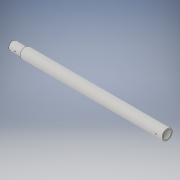
# Autodesk Inventor part: 1_6RadiusPoleAJB
Saved by Autodesk Inventor 2018 (Build 220112000, 112)
## iProperties
Created: 2018-02-02
Part Number: 1_6RadiusPoleAJB
Material: Generic
Document SubType Name: Modeling
Designer: Alec temporary
Density: 1 g/cm^3
Appearance: Default
Author: Alec temporary
Autodesk Inventor part; units mm, degrees
ref_plane "YZ Plane" through (0, 0, 0) normal (1, 0, 0) x (0, 1, 0)
ref_plane "XZ Plane" through (0, 0, 0) normal (0, 1, 0) x (-1, 0, 0)
sketch "Sketch1" plane through (0, 0, 0) normal (0, 0, 1) x (1, 0, 0)
  circle A0 centre (0, 0) radius 22860 construction
  line L0 (0, 127) -> (0, -127)
  line L1 (0, -127) -> (-22859.6472, -127) construction
  line L2 (-22859.6472, -127) -> (-22859.6472, 127) construction
  line L3 (-22859.6472, 127) -> (0, 127) construction
  line L4 (0, 0) -> (-22859.6472, 0) construction
  line L5 (0, 127) -> (-3809.9412, 127)
  line L6 (-3809.9412, 127) -> (-3809.9412, -127)
  line L7 (-3809.9412, -127) -> (0, -127)
  dimension "d0" = 45720
  dimension "d1" = 254
  dimension "d2" = 22859.6472
  dimension "d3" = 3809.9412
  constraints: 16 end point, 2 coincident, 2 midpoint, 2 parallel, 2 point on circle, 2 point on line, 1 centre point, 1 collinear, 1 perpendicular, 1 vertical
  measures "d0" diameter of A0
  measures "d1" distance of L0.start L0.end
  measures "d2" distance of L4.start L4.end
  measures "d3" distance of L6.end L0.end
extrude "Main Extursion" add sketch "Sketch1" along normal mid plane 254
fillet "Fillet1" radius 127 4 edges at (-1904.9706, 127, 127) (-1904.9706, -127, -127) (-1904.9706, -127, 127) (-1904.9706, 127, -127)
sketch "Sketch2" plane through (0, 0, 0) normal (1, 0, 0) x (0, 0, -1)
  circle A0 centre (0, 0) radius 101.6
  dimension "d7" = 203.2
  constraints: 1 centre point, 1 coincident
  measures "d7" diameter of A0
extrude "Female" cut sketch "Sketch2" against normal blind 304.8
ref_plane "Work Plane1" through (-952.4853, 0, 127) normal (0, 0, 1) x (1, 0, 0)
sketch "Sketch3" plane through (-3809.9412, 0, 0) normal (-1, 0, 0) x (0, 0, 1)
  circle A0 centre (0, 0) radius 101.6
  circle A1 centre (0, 0) radius 127 projected
  dimension "d10" = 203.2
  constraints: 1 centre point, 1 coincident
  measures "d10" diameter of A0
extrude "Male" cut sketch "Sketch3" against normal blind 304.8
sketch "Sketch4" plane through (0, 0, 127) normal (0, 0, 1) x (1, 0, 0)
  circle A0 centre (-3657.5412, 0) radius 12.7
  circle A1 centre (-152.4, 0) radius 12.7
  line L0 (-3809.9412, 101.6) -> (-3809.9412, -101.6) projected
  point P0 (0, 0)
  dimension "d13" = 25.4
  dimension "d14" = 25.4
  dimension "d15" = 152.4
  dimension "d16" = 152.4
  constraints: 2 centre point, 2 horizontal alignment
  measures "d13" diameter of A1
  measures "d14" diameter of A0
  measures "d15" distance from line of L0 A0.centre
  measures "d16" distance of point (0, 0) A1.centre
hole "BoltHole" at (-3657.5412, 0, 127) at (-152.4, 0, 127) direction (0, 0, -1) diameter 21.971 end through all thread size "1-8 UNC" class "2B" standard "ANSI Unified Screw Threads"
equation "\"d3\" = 0.166667 * d2"
equation "\"d14\" = d13"
body "Solid1"
